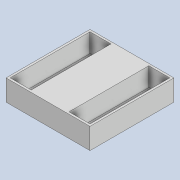
# Autodesk Inventor part: Box
Saved by Autodesk Inventor 2021 (Build 250183000, 183)
## iProperties
Created: 2021-06-04
Part Number: Box
Material: Generic
Document SubType Name: Modeling
Designer: CAROLINA
Density: 1 g/cm^3
Appearance: Default
Author: CAROLINA
Autodesk Inventor part; units mm, degrees
ref_plane "YZ Plane" through (0, 0, 0) normal (1, 0, 0) x (0, 1, 0)
ref_plane "XZ Plane" through (0, 0, 0) normal (0, 1, 0) x (-1, 0, 0)
ref_plane "XY Plane" through (0, 0, 0) normal (0, 0, 1) x (1, 0, 0)
sketch "Sketch1" plane through (0, 0, 0) normal (0, 1, 0) x (-1, 0, 0)
  line L0 (0, 0) -> (200, 0)
  line L1 (200, 0) -> (200, -200)
  line L2 (200, -200) -> (0, -200)
  line L3 (0, -200) -> (0, 0)
  dimension "d0" = 200
  dimension "d1" = 200
  constraints: 8 end point, 2 parallel, 1 horizontal, 1 perpendicular
  measures "d0" distance of L1.end L2.end
  measures "d1" distance of L0.end L1.end
extrude "Extrusion1" add sketch "Sketch1" along normal blind 50
sketch "Sketch2" plane through (0, 50, 0) normal (0, 1, 0) x (1, 0, 0)
  line L0 (-5, 5) -> (-5, 195)
  line L1 (0, 200) -> (-200, 200) projected
  line L2 (-5, 195) -> (-55, 195)
  line L3 (-55, 195) -> (-55, 5)
  line L4 (-55, 5) -> (-5, 5)
  line L5 (-200, 200) -> (-200, 0) projected
  line L6 (-195, 195) -> (-145, 195)
  line L7 (-145, 195) -> (-145, 5)
  line L8 (-145, 5) -> (-195, 5)
  line L9 (-195, 5) -> (-195, 195)
  point P0 (0, 0)
  dimension "d4" = 190
  dimension "d5" = 50
  dimension "d16" = 50
  dimension "d17" = 190
  dimension "d20" = 5
  constraints: 16 end point, 5 perpendicular, 2 parallel, 1 horizontal
  measures "d4" distance of L0.start L0.end
  measures "d5" distance of L0.end L2.end
  measures "d16" distance of L7.end L8.end
  measures "d17" distance of L6.end L7.end
  measures "d20" distance between parallel lines of L5 L9
extrude "Extrusion2" cut sketch "Sketch2" against normal blind 45 contours L4 L3 L2 L0
extrude "Extrusión4" cut sketch "Sketch2" against normal blind 45 contours L6 L7 L8 L9
body "Solid1"
